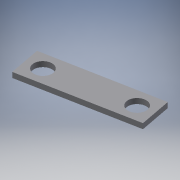
# Autodesk Inventor part: LeverArm
Saved by Autodesk Inventor 2018 (Build 220112000, 112)
## iProperties
Created: 2018-05-20
Part Number: LeverArm
Material: Generic
Document SubType Name: Modeling
Designer: reide
Density: 1 g/cm^3
Appearance: Default
Author: reide
Autodesk Inventor part; units mm, degrees
ref_plane "YZ Plane" through (0, 0, 0) normal (1, 0, 0) x (0, 1, 0)
ref_plane "XZ Plane" through (0, 0, 0) normal (0, 1, 0) x (-1, 0, 0)
ref_plane "XY Plane" through (0, 0, 0) normal (0, 0, 1) x (1, 0, 0)
sketch "Sketch1" plane through (0, 0, 0) normal (0, 0, 1) x (1, 0, 0)
  line L0 (-12.5, -2.5) -> (-12.5, 2.5) projected
  line L1 (-12.5, 2.5) -> (-17.5, 2.5) projected
  line L2 (-17.5, 2.5) -> (-17.5, 7.5) projected
  line L3 (-32.5, 7.5) -> (-17.5, 7.5) projected
  arc A0 (-32.5, 7.5) -> (-12.5, -2.5) centre (-12.5, 22.5) ccw projected
  circle A1 centre (-22.5, 4) radius 1.75
  circle A2 centre (-37.6776, 1.0985) radius 1.75
  line L4 (-22.5, 4) -> (-37.6776, 1.0985)
  line L5 (-22.5, 4) -> (-21.7788, 0.2278)
  line L6 (-22.5, 4) -> (-21.9367, 1.0534)
  line L7 (-37.6776, 1.0985) -> (-37.1143, -1.8482)
  line L8 (-21.9367, 1.0534) -> (-37.1143, -1.8482)
  line L9 (-22.5, 4) -> (-19.5534, 4.5633)
  line L10 (-21.9367, 1.0534) -> (-18.99, 1.6167)
  line L11 (-18.99, 1.6167) -> (-19.5534, 4.5633)
  line L12 (-37.6776, 1.0985) -> (-38.2409, 4.0451)
  line L13 (-23.0633, 6.9466) -> (-38.2409, 4.0451)
  line L14 (-23.0633, 6.9466) -> (-20.1167, 7.51)
  line L15 (-20.1167, 7.51) -> (-19.5534, 4.5633)
  line L16 (-37.1143, -1.8482) -> (-40.0609, -2.4115)
  line L17 (-40.0609, -2.4115) -> (-41.1875, 3.4818)
  line L18 (-41.1875, 3.4818) -> (-38.2409, 4.0451)
  line L19 (-18.99, 1.6167) -> (-40.0609, -2.4115)
  line L20 (-40.0609, -2.4115) -> (-41.1875, 3.4818)
  line L21 (-41.1875, 3.4818) -> (-20.1167, 7.51)
  point P0 (0, 0)
  dimension "d0" = 3.5
  dimension "d1" = 3.5
  dimension "d2" = 90
  dimension "d3" = 3
  dimension "d4" = 3
  dimension "d5" = 180
  dimension "d6" = 3
  constraints: 36 end point, 3 perpendicular, 3 symmetric about line, 2 centre point, 2 collinear, 2 point on line
  measures "d0" diameter of A1
  measures "d1" diameter of A2
  measures "d2" angle of L4 L5
  measures "d3" distance of L4.start L6.end
  measures "d4" distance of L4.start L9.end
  measures "d5" angle of L4 L9
  measures "d6" distance of L7.end L16.end
extrude "Extrusion1" add sketch "Sketch1" along normal blind 1 contours L8 L7 A2 L4 A0 | A0 L4 A1 L5 L8 | L4 A2 L12 L13 A0 | A0 L13 L14 L3 L15 L9 A1 L4 | L5 A1 L9 L11 L10 | L16 L17 L18 L12 A2 L7 | L4 L5 A1 | L4 L12 A2 | A2 L7 L4 | L5 L9 A1 | A2 L12 L7 | L3 L14 L15
sketch "Sketch2" plane through (0, 0, 1) normal (0, 0, 1) x (1, 0, 0)
  arc A0 (-20.7811, 4.3286) -> (-24.2189, 3.6714) centre (-22.5, 4) ccw projected
  line L0 (-68.111, -8.1624) -> (-72.0972, 25.6031) projected
  line L1 (-29.38, -3.59) -> (-68.111, -8.1624) projected
  line L2 (-33.3662, 30.1755) -> (-29.38, -3.59) projected
  line L3 (-72.0972, 25.6031) -> (-33.3662, 30.1755) projected
  line L4 (-24.2189, 3.6714) -> (-20.7811, 4.3286) projected
  circle A1 centre (-22.5, 4) radius 1.75
  line L5 (-37.6776, 1.0985) -> (-35.9587, 1.4271) projected
  circle A2 centre (-37.6776, 1.0985) radius 1.75
  point P0 (0, 0)
  constraints: 1 coincident, 6 other
extrude "Extrusion2" cut sketch "Sketch2" against normal blind 1 contours L4 A0 | A1 L4 | A2
fillet "Fillet1" radius 1 4 edges at (-40.0609, -2.4115, 0.5) (-41.1875, 3.4818, 0.5) (-18.99, 1.6167, 0.5) (-20.1167, 7.51, 0.5)
body "Solid1"
